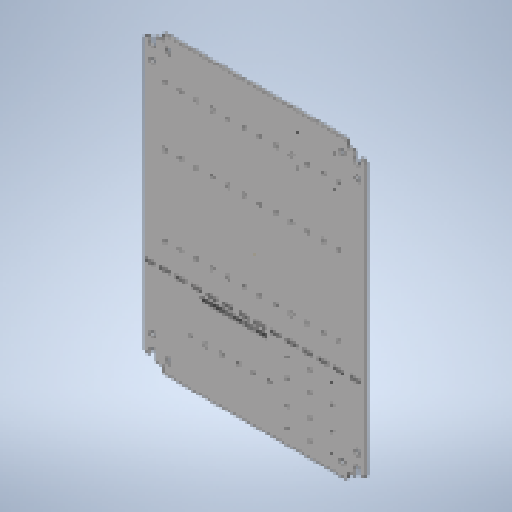
# Autodesk Inventor part: assembly-board
Saved by Autodesk Inventor 2023 (Build 270158030, 158C)
## iProperties
Created: 2024-03-20
Part Number: assembly-board
Material: Generic
Document SubType Name: Modeling
Designer: Imogen Heard
Density: 1 g/cm^3
Appearance: Default
Author: Imogen Heard
Autodesk Inventor part; units mm, degrees
(part 1 of 2)
ref_plane "YZ Plane" through (0, 0, 0) normal (1, 0, 0) x (0, 1, 0)
ref_plane "XZ Plane" through (0, 0, 0) normal (0, 1, 0) x (-1, 0, 0)
ref_plane "XY Plane" through (0, 0, 0) normal (0, 0, 1) x (1, 0, 0)
sketch "high voltage" plane through (0, 0, 0) normal (0, 0, 1) x (1, 0, 0)
  line L0 (-121.4929, -169.2156) -> (-167.7133, -169.2156)
  line L1 (-169.4454, -166.2156) -> (-146.3352, -126.1875)
  line L2 (-142.8711, -126.1875) -> (-119.7608, -166.2156)
  arc A0 (-142.8711, -126.1875) -> (-146.3352, -126.1875) centre (-144.6031, -127.1875) ccw
  arc A1 (-169.4454, -166.2156) -> (-167.7133, -169.2156) centre (-167.7133, -167.2156) ccw
  arc A2 (-121.4929, -169.2156) -> (-119.7608, -166.2156) centre (-121.4929, -167.2156) ccw
  line L3 (-145.4691, -126.6875) -> (-168.5793, -166.7156)
  arc A3 (-168.5793, -166.7156) -> (-167.7133, -168.2156) centre (-167.7133, -167.2156) ccw
  line L4 (-167.7133, -168.2156) -> (-121.4929, -168.2156)
  arc A4 (-121.4929, -168.2156) -> (-120.6269, -166.7156) centre (-121.4929, -167.2156) ccw
  line L5 (-120.6269, -166.7156) -> (-143.7371, -126.6875)
  arc A5 (-143.7371, -126.6875) -> (-145.4691, -126.6875) centre (-144.6031, -127.1875) ccw
  line L6 (-146.1782, -139.2847) -> (-142.8711, -139.2847)
  line L7 (-142.8711, -139.2847) -> (-147.4472, -150.1934)
  line L8 (-147.4472, -150.1934) -> (-140.7016, -147.4551)
  line L9 (-140.7016, -147.4551) -> (-144.0744, -160.167)
  line L10 (-144.0744, -160.167) -> (-142.8711, -160.167)
  line L11 (-142.8711, -160.167) -> (-145.822, -164.4859)
  line L12 (-145.822, -164.4859) -> (-147.4472, -160.0557)
  line L13 (-147.4472, -160.0557) -> (-146.1782, -160.0557)
  line L14 (-146.1782, -160.0557) -> (-143.8332, -151.8141)
  line L15 (-143.8332, -151.8141) -> (-150.3785, -154.471)
  line L16 (-150.3785, -154.471) -> (-146.1782, -139.2847)
  point P0 (-144.8622, -153.6861)
  point P1 (-144.6031, -153.8729)
  point P2 (-144.6031, -153.8729)
  point P3 (-118.0288, -169.2156)
  point P4 (-171.1774, -169.2156)
  point P5 (-144.6031, -123.1875)
  dimension "d142" = 2
  dimension "d146" = 1
  measures "d142" radius of A0
  measures "d146" distance between parallel lines of L3 L1
sketch "Sketch1" plane through (0, 0, 0) normal (0, 0, 1) x (1, 0, 0)
  line L0 (-175, 232.5) -> (175, 232.5)
  line L1 (175, 232.5) -> (175, -232.5)
  line L2 (175, -232.5) -> (-175, -232.5)
  line L3 (-175, -232.5) -> (-175, 232.5)
  point P0 (0, 0)
  dimension "d0" = 350
  dimension "d1" = 465
  dimension "d2" = 232.5
  dimension "d3" = 175
  constraints: 8 end point, 2 parallel, 1 horizontal, 1 perpendicular
  measures "d0" distance between parallel lines of L1 L3
  measures "d1" distance between parallel lines of L2 L0
  measures "d2" distance from line of point (0, 0) L0
  measures "d3" distance from line of point (0, 0) L1
extrude "Extrusion1" add sketch "Sketch1" along normal blind 3
sketch "Sketch3" plane through (0, 0, 3) normal (0, 0, 1) x (1, 0, 0)
  line L0 (-175, -232.5) -> (175, -232.5) projected
  line L1 (175, 232.5) -> (-175, 232.5) projected
  line L2 (175, -232.5) -> (175, 232.5) projected
  line L3 (-175, 232.5) -> (-175, -232.5) projected
  line L4 (-175, 232.5) -> (-146.5, 232.5)
  line L5 (-146.5, 232.5) -> (-146.5, 222.5)
  line L6 (-146.5, 222.5) -> (-175, 222.5)
  line L7 (-175, 222.5) -> (-175, 232.5)
  line L8 (-156, 216.5) -> (-175, 216.5)
  line L9 (-175, 216.5) -> (-175, 222.5)
  line L10 (-175, 222.5) -> (-156, 222.5)
  line L11 (-156, 222.5) -> (-156, 216.5)
  line L12 (-156, 216.5) -> (-167, 216.5)
  line L13 (-167, 216.5) -> (-167, 211.5)
  line L14 (-167, 211.5) -> (-156, 211.5)
  line L15 (-156, 211.5) -> (-156, 216.5)
  arc A0 (-167, 211.5) -> (-156, 211.5) centre (-161.5, 211.5) ccw
  line L16 (-146.5, 229.5) -> (-143.5, 232.5)
  line L17 (-175, 213.5) -> (-172, 216.5)
  circle A1 centre (-162, 187) radius 4.2
  circle A2 centre (-137.5, 211.5) radius 4.2
  point P0 (0, 0)
  dimension "d7" = 465
  dimension "d8" = 350
  dimension "d9" = 28.5
  dimension "d10" = 10
  dimension "d11" = 6
  dimension "d12" = 19
  dimension "d14" = 5
  dimension "d15" = 11
  dimension "d16" = 45
  dimension "d17" = 3
  dimension "d18" = 3
  dimension "d19" = 45
  dimension "d22" = 8.4
  dimension "d23" = 13
  dimension "d24" = 13.5
  dimension "d25" = 45.5
  dimension "d26" = 37.5
  dimension "d27" = 21
  constraints: 28 end point, 6 parallel, 3 centre point, 3 horizontal, 3 perpendicular, 3 point on line, 2 coincident, 2 point on circle, 1 equal radius, 1 horizontal alignment, 1 midpoint
  measures "d7" distance between parallel lines of L0 L1
  measures "d8" distance between parallel lines of L2 L3
  measures "d9" distance between parallel lines of L3 L5
  measures "d10" distance between parallel lines of L6 L1
  measures "d11" distance between parallel lines of L8 L6
  measures "d12" distance between parallel lines of L3 L11
  measures "d14" distance between parallel lines of L14 L12
  measures "d15" distance between parallel lines of L13 L15
  measures "d16" angle of L5 L16
  measures "d17" distance of L4.end L16.end
  measures "d18" distance from line of L3 L17.end
  measures "d19" angle of L8 L17
  measures "d22" diameter of A2
  measures "d23" distance from line of L3 A1.centre
  measures "d24" distance from line of L3 A0.centre
  measures "d25" distance from line of A1.centre L1
  measures "d26" distance from line of A2.centre L3
  measures "d27" distance from line of L1 A2.centre
extrude "Extrusion2" cut sketch "Sketch3" against normal through all contours L3 L8 L17 | L3 L6 L11 L8 | L16 L5 L1 | L3 L1 L5 L6 | L8 L15 L14 L13 | L14 A0 | A1 | A2
mirror "Mirror1" about plane through (0, 0, 0) normal (1, 0, 0) of "Extrusion2"
mirror "Mirror2" about plane through (0, 0, 0) normal (0, 1, 0) of "Extrusion2", "Mirror1"
sketch "Sketch4" plane through (0, 0, 3) normal (0, 0, 1) x (1, 0, 0)
  circle A0 centre (66.2112, 202.7338) radius 1.35 projected
  circle A1 centre (124.2112, 202.7338) radius 1.35 projected
  circle A2 centre (124.2112, 153.7338) radius 1.35 projected
  circle A3 centre (66.2112, 153.7338) radius 1.35 projected
  circle A4 centre (-142.425, 75.1905) radius 2.6
  arc A5 (113.375, 71.9905) -> (113.375, 78.3905) centre (113.375, 75.1905) ccw projected
  line L0 (113.375, 71.9905) -> (101.775, 71.9905) projected
  arc A6 (101.775, 78.3905) -> (101.775, 71.9905) centre (101.775, 75.1905) ccw projected
  line L1 (101.775, 78.3905) -> (113.375, 78.3905) projected
  arc A7 (-111.625, 71.9905) -> (-111.625, 78.3905) centre (-111.625, 75.1905) ccw projected
  line L2 (-111.625, 71.9905) -> (-123.225, 71.9905) projected
  arc A8 (-123.225, 78.3905) -> (-123.225, 71.9905) centre (-123.225, 75.1905) ccw projected
  line L3 (-123.225, 78.3905) -> (-111.625, 78.3905) projected
  arc A9 (13.375, 71.9905) -> (13.375, 78.3905) centre (13.375, 75.1905) ccw projected
  line L4 (13.375, 71.9905) -> (1.775, 71.9905) projected
  arc A10 (1.775, 78.3905) -> (1.775, 71.9905) centre (1.775, 75.1905) ccw projected
  line L5 (1.775, 78.3905) -> (13.375, 78.3905) projected
  arc A11 (-11.625, 71.9905) -> (-11.625, 78.3905) centre (-11.625, 75.1905) ccw projected
  line L6 (-11.625, 71.9905) -> (-23.225, 71.9905) projected
  arc A12 (-23.225, 78.3905) -> (-23.225, 71.9905) centre (-23.225, 75.1905) ccw projected
  line L7 (-23.225, 78.3905) -> (-11.625, 78.3905) projected
  arc A13 (-86.625, 71.9905) -> (-86.625, 78.3905) centre (-86.625, 75.1905) ccw projected
  line L8 (-86.625, 71.9905) -> (-98.225, 71.9905) projected
  arc A14 (-98.225, 78.3905) -> (-98.225, 71.9905) centre (-98.225, 75.1905) ccw projected
  line L9 (-98.225, 78.3905) -> (-86.625, 78.3905) projected
  arc A15 (88.375, 71.9905) -> (88.375, 78.3905) centre (88.375, 75.1905) ccw projected
  line L10 (88.375, 71.9905) -> (76.775, 71.9905) projected
  arc A16 (76.775, 78.3905) -> (76.775, 71.9905) centre (76.775, 75.1905) ccw projected
  line L11 (76.775, 78.3905) -> (88.375, 78.3905) projected
  arc A17 (138.375, 71.9905) -> (138.375, 78.3905) centre (138.375, 75.1905) ccw projected
  line L12 (138.375, 71.9905) -> (126.775, 71.9905) projected
  arc A18 (126.775, 78.3905) -> (126.775, 71.9905) centre (126.775, 75.1905) ccw projected
  line L13 (126.775, 78.3905) -> (138.375, 78.3905) projected
  arc A19 (-61.625, 71.9905) -> (-61.625, 78.3905) centre (-61.625, 75.1905) ccw projected
  line L14 (-61.625, 71.9905) -> (-73.225, 71.9905) projected
  arc A20 (-73.225, 78.3905) -> (-73.225, 71.9905) centre (-73.225, 75.1905) ccw projected
  line L15 (-73.225, 78.3905) -> (-61.625, 78.3905) projected
  arc A21 (38.375, 71.9905) -> (38.375, 78.3905) centre (38.375, 75.1905) ccw projected
  line L16 (38.375, 71.9905) -> (26.775, 71.9905) projected
  arc A22 (26.775, 78.3905) -> (26.775, 71.9905) centre (26.775, 75.1905) ccw projected
  line L17 (26.775, 78.3905) -> (38.375, 78.3905) projected
  arc A23 (-36.625, 71.9905) -> (-36.625, 78.3905) centre (-36.625, 75.1905) ccw projected
  line L18 (-36.625, 71.9905) -> (-48.225, 71.9905) projected
  arc A24 (-48.225, 78.3905) -> (-48.225, 71.9905) centre (-48.225, 75.1905) ccw projected
  line L19 (-48.225, 78.3905) -> (-36.625, 78.3905) projected
  line L20 (-148.225, 78.3905) -> (-136.625, 78.3905) projected
  arc A25 (-136.625, 71.9905) -> (-136.625, 78.3905) centre (-136.625, 75.1905) ccw projected
  line L21 (-136.625, 71.9905) -> (-148.225, 71.9905) projected
  arc A26 (-148.225, 78.3905) -> (-148.225, 71.9905) centre (-148.225, 75.1905) ccw projected
  arc A27 (63.375, 71.9905) -> (63.375, 78.3905) centre (63.375, 75.1905) ccw projected
  line L22 (63.375, 71.9905) -> (51.775, 71.9905) projected
  arc A28 (51.775, 78.3905) -> (51.775, 71.9905) centre (51.775, 75.1905) ccw projected
  line L23 (51.775, 78.3905) -> (63.375, 78.3905) projected
  line L24 (-155.025, 86.8905) -> (-155.025, 63.4905) projected
  line L25 (-155.025, 63.4905) -> (144.975, 63.4905) projected
  line L26 (144.975, 86.8905) -> (144.975, 63.4905) projected
  line L27 (-155.025, 86.8905) -> (144.975, 86.8905) projected
  circle A29 centre (-117.425, 75.1905) radius 2.6
  circle A30 centre (-92.425, 75.1905) radius 2.6
  circle A31 centre (-67.425, 75.1905) radius 2.6
  circle A32 centre (-42.425, 75.1905) radius 2.6
  circle A33 centre (-17.425, 75.1905) radius 2.6
  circle A34 centre (7.575, 75.1905) radius 2.6
  circle A35 centre (32.575, 75.1905) radius 2.6
  circle A36 centre (57.575, 75.1905) radius 2.6
  circle A37 centre (82.575, 75.1905) radius 2.6
  circle A38 centre (107.575, 75.1905) radius 2.6
  circle A39 centre (132.575, 75.1905) radius 2.6
  circle A40 centre (-142.425, -49.8095) radius 2.6
  circle A41 centre (-117.425, -49.8095) radius 2.6
  circle A42 centre (-92.425, -49.8095) radius 2.6
  circle A43 centre (-67.425, -49.8095) radius 2.6
  circle A44 centre (-42.425, -49.8095) radius 2.6
  circle A45 centre (-17.425, -49.8095) radius 2.6
  circle A46 centre (7.575, -49.8095) radius 2.6
  circle A47 centre (32.575, -49.8095) radius 2.6
  circle A48 centre (57.575, -49.8095) radius 2.6
  circle A49 centre (82.575, -49.8095) radius 2.6
  circle A50 centre (107.575, -49.8095) radius 2.6
  circle A51 centre (132.575, -49.8095) radius 2.6
  line L28 (24.975, -156.6095) -> (24.975, -148.1095) projected
  line L29 (-115.025, -148.1095) -> (24.975, -148.1095) projected
  line L30 (-115.025, -148.1095) -> (-115.025, -171.5095) projected
  line L31 (-115.025, -171.5095) -> (24.975, -171.5095) projected
  line L32 (24.975, -171.5095) -> (24.975, -163.0095) projected
  line L33 (24.975, -163.0095) -> (16.775, -163.0095) projected
  arc A52 (16.775, -156.6095) -> (16.775, -163.0095) centre (16.775, -159.8095) ccw projected
  line L34 (16.775, -156.6095) -> (24.975, -156.6095) projected
  arc A53 (-71.625, -163.0095) -> (-71.625, -156.6095) centre (-71.625, -159.8095) ccw projected
  line L35 (-71.625, -163.0095) -> (-83.225, -163.0095) projected
  arc A54 (-83.225, -156.6095) -> (-83.225, -163.0095) centre (-83.225, -159.8095) ccw projected
  line L36 (-83.225, -156.6095) -> (-71.625, -156.6095) projected
  arc A55 (-46.625, -163.0095) -> (-46.625, -156.6095) centre (-46.625, -159.8095) ccw projected
  line L37 (-46.625, -163.0095) -> (-58.225, -163.0095) projected
  arc A56 (-58.225, -156.6095) -> (-58.225, -163.0095) centre (-58.225, -159.8095) ccw projected
  line L38 (-58.225, -156.6095) -> (-46.625, -156.6095) projected
  arc A57 (-21.625, -163.0095) -> (-21.625, -156.6095) centre (-21.625, -159.8095) ccw projected
  line L39 (-21.625, -163.0095) -> (-33.225, -163.0095) projected
  arc A58 (-33.225, -156.6095) -> (-33.225, -163.0095) centre (-33.225, -159.8095) ccw projected
  line L40 (-33.225, -156.6095) -> (-21.625, -156.6095) projected
  arc A59 (3.375, -163.0095) -> (3.375, -156.6095) centre (3.375, -159.8095) ccw projected
  line L41 (3.375, -163.0095) -> (-8.225, -163.0095) projected
  arc A60 (-8.225, -156.6095) -> (-8.225, -163.0095) centre (-8.225, -159.8095) ccw projected
  line L42 (-8.225, -156.6095) -> (3.375, -156.6095) projected
  line L43 (-108.225, -156.6095) -> (-96.625, -156.6095) projected
  arc A61 (-96.625, -163.0095) -> (-96.625, -156.6095) centre (-96.625, -159.8095) ccw projected
  line L44 (-96.625, -163.0095) -> (-108.225, -163.0095) projected
  arc A62 (-108.225, -156.6095) -> (-108.225, -163.0095) centre (-108.225, -159.8095) ccw projected
  circle A63 centre (-102.425, -159.8095) radius 2.6
  circle A64 centre (-77.425, -159.8095) radius 2.6
  circle A65 centre (-52.425, -159.8095) radius 2.6
  circle A66 centre (-27.425, -159.8095) radius 2.6
  circle A67 centre (-2.425, -159.8095) radius 2.6
  circle A68 centre (22.575, -159.8095) radius 2.6
  arc A69 (49.282, -111.3926) -> (52.922, -111.3926) centre (51.102, -111.3926) ccw projected
  arc A70 (84.282, -111.3926) -> (87.922, -111.3926) centre (86.102, -111.3926) ccw projected
  arc A71 (119.282, -111.3926) -> (122.922, -111.3926) centre (121.102, -111.3926) ccw projected
  circle A72 centre (121.102, -142.2926) radius 1.82 projected
  circle A73 centre (86.102, -142.2926) radius 1.82 projected
  circle A74 centre (51.102, -142.2926) radius 1.82 projected
  circle A75 centre (51.102, -178.1926) radius 1.82 projected
  circle A76 centre (86.102, -178.1926) radius 1.82 projected
  circle A77 centre (121.102, -178.1926) radius 1.82 projected
  arc A78 (122.922, -209.0926) -> (119.282, -209.0926) centre (121.102, -209.0926) ccw projected
  arc A79 (87.922, -209.0926) -> (84.282, -209.0926) centre (86.102, -209.0926) ccw projected
  arc A80 (52.922, -209.0926) -> (49.282, -209.0926) centre (51.102, -209.0926) ccw projected
  circle A81 centre (51.102, -209.0926) radius 1.6
  circle A82 centre (86.102, -209.0926) radius 1.6
  circle A83 centre (121.102, -209.0926) radius 1.6
  circle A84 centre (51.102, -111.5926) radius 1.6
  circle A85 centre (86.102, -111.5926) radius 1.6
  circle A86 centre (121.102, -111.5926) radius 1.6
  circle A87 centre (-142.425, 167.1905) radius 2.6
  circle A88 centre (-117.425, 75.1905) radius 2.6
  circle A89 centre (-117.425, 167.1905) radius 2.6
  circle A90 centre (-92.425, 75.1905) radius 2.6
  circle A91 centre (-92.425, 167.1905) radius 2.6
  circle A92 centre (-67.425, 75.1905) radius 2.6
  circle A93 centre (-67.425, 167.1905) radius 2.6
  circle A94 centre (-42.425, 75.1905) radius 2.6
  circle A95 centre (-42.425, 167.1905) radius 2.6
  circle A96 centre (-17.425, 75.1905) radius 2.6
  circle A97 centre (-17.425, 167.1905) radius 2.6
  circle A98 centre (7.575, 75.1905) radius 2.6
  circle A99 centre (7.575, 167.1905) radius 2.6
  circle A100 centre (32.575, 75.1905) radius 2.6
  circle A101 centre (32.575, 167.1905) radius 2.6
  circle A102 centre (57.575, 75.1905) radius 2.6
  circle A103 centre (57.575, 167.1905) radius 2.6
  circle A104 centre (82.575, 75.1905) radius 2.6
  circle A105 centre (82.575, 167.1905) radius 2.6
  circle A106 centre (107.575, 75.1905) radius 2.6
  circle A107 centre (107.575, 167.1905) radius 2.6
  circle A108 centre (132.575, 75.1905) radius 2.6
  circle A109 centre (132.575, 167.1905) radius 2.6
  point P0 (0, 0)
  dimension "d28" = 5.2
  dimension "d29" = 5.8
  dimension "d30" = 5.8
  dimension "d31" = 25
  dimension "d34" = 25
  dimension "d37" = 125
  dimension "d40" = 5.2
  dimension "d41" = 5.8
  dimension "d44" = 25
  dimension "d49" = 3.2
  dimension "d52" = 35
  dimension "d55" = 97.5
  dimension "d60" = 92
  dimension "d63" = 25
  constraints: 59 centre point, 4 horizontal, 3 vertical, 2 horizontal alignment, 1 coincident, 112 other
  measures "d28" diameter of A4
  measures "d29" distance of A26.centre A4.centre
  measures "d30" distance of A25.centre A4.centre
  measures "d31" distance of A7.centre A25.centre
  measures "d34" distance of A4.centre A29.centre
  measures "d37" distance of A4.centre A40.centre
  measures "d40" diameter of A63
  measures "d41" distance of A62.centre A63.centre
  measures "d44" distance of A63.centre A64.centre
  measures "d49" diameter of A81
  measures "d52" distance of A81.centre A82.centre
  measures "d55" distance of A81.centre A84.centre
  measures "d60" distance of A4.centre A87.centre
  measures "d63" distance of A4.centre A88.centre
extrude "Extrusion3" cut sketch "Sketch4" against normal through all contours A0 | A1 | A2 | A3 | A4 | A29 | A30 | A31 | A32 | A33 | A34 | A35 | A36 | A37 | A38 | A39 | A40 | A41 | A42 | A43 | A44 | A45 | A46 | A47 | A48 | A49 | A50 | A51 | A63 | A64 | A65 | A66 | A67 | A68 | A72 | A73 | A74 | A75 | A76 | A77 | A81 | A82 | A83 | A84 | A85 | A86 | A87 | A89 | A91 | A93 | A95 | A97 | A99 | A101 | A103 | A105 | A107 | A109
sketch "Sketch5" plane through (0, 0, 3) normal (0, 0, 1) x (1, 0, 0)
  line L0 (-175, 213.5) -> (-175, -213.5) projected
  line L1 (-175, -87.5) -> (-160, -87.5)
  line L2 (-160, -87.5) -> (-160, -91.5)
  line L3 (-160, -91.5) -> (-175, -91.5)
  line L4 (-175, -91.5) -> (-175, -87.5)
  line L5 (-143.5, -232.5) -> (143.5, -232.5) projected
  line L6 (-150, -87.5) -> (-135, -87.5)
  line L7 (-135, -91.5) -> (-150, -91.5)
  line L8 (-135, -87.5) -> (-135, -91.5)
  line L9 (-150, -91.5) -> (-150, -87.5)
  line L10 (-125, -87.5) -> (-110, -87.5)
  line L11 (-110, -91.5) -> (-125, -91.5)
  line L12 (-110, -87.5) -> (-110, -91.5)
  line L13 (-125, -91.5) -> (-125, -87.5)
  line L14 (-100, -87.5) -> (-85, -87.5)
  line L15 (-85, -91.5) -> (-100, -91.5)
  line L16 (-85, -87.5) -> (-85, -91.5)
  line L17 (-100, -91.5) -> (-100, -87.5)
  line L18 (-75, -87.5) -> (-60, -87.5)
  line L19 (-60, -91.5) -> (-75, -91.5)
  line L20 (-60, -87.5) -> (-60, -91.5)
  line L21 (-75, -91.5) -> (-75, -87.5)
  line L22 (-50, -87.5) -> (-35, -87.5)
  line L23 (-35, -91.5) -> (-50, -91.5)
  line L24 (-35, -87.5) -> (-35, -91.5)
  line L25 (-50, -91.5) -> (-50, -87.5)
  line L26 (-25, -87.5) -> (-10, -87.5)
  line L27 (-10, -91.5) -> (-25, -91.5)
  line L28 (-10, -87.5) -> (-10, -91.5)
  line L29 (-25, -91.5) -> (-25, -87.5)
  line L30 (0, -87.5) -> (15, -87.5)
  line L31 (15, -91.5) -> (0, -91.5)
  line L32 (15, -87.5) -> (15, -91.5)
  line L33 (0, -91.5) -> (0, -87.5)
  line L34 (25, -87.5) -> (40, -87.5)
  line L35 (40, -91.5) -> (25, -91.5)
  line L36 (40, -87.5) -> (40, -91.5)
  line L37 (25, -91.5) -> (25, -87.5)
  line L38 (50, -87.5) -> (65, -87.5)
  line L39 (65, -91.5) -> (50, -91.5)
  line L40 (65, -87.5) -> (65, -91.5)
  line L41 (50, -91.5) -> (50, -87.5)
  line L42 (75, -91.5) -> (75, -87.5)
  line L43 (90, -91.5) -> (75, -91.5)
  line L44 (90, -87.5) -> (90, -91.5)
  line L45 (75, -87.5) -> (90, -87.5)
  line L46 (100, -91.5) -> (100, -87.5)
  line L47 (115, -91.5) -> (100, -91.5)
  line L48 (115, -87.5) -> (115, -91.5)
  line L49 (100, -87.5) -> (115, -87.5)
  line L50 (125, -91.5) -> (125, -87.5)
  line L51 (140, -91.5) -> (125, -91.5)
  line L52 (140, -87.5) -> (140, -91.5)
  line L53 (125, -87.5) -> (140, -87.5)
  line L54 (150, -91.5) -> (150, -87.5)
  line L55 (165, -91.5) -> (150, -91.5)
  line L56 (165, -87.5) -> (165, -91.5)
  line L57 (150, -87.5) -> (165, -87.5)
  line L58 (-84.5169, -96.4994) -> (24.8633, -96.4994) construction
  line L59 (24.8633, -96.4994) -> (24.8633, -107.8996) construction
  line L60 (24.8633, -107.8996) -> (-84.5169, -107.8996) construction
  line L61 (-84.5169, -107.8996) -> (-84.5169, -96.4994) construction
  line L62 (-67.4562, -118.0258) -> (-47.9562, -118.0258)
  line L63 (-47.9562, -118.0258) -> (-47.9562, -203.2928)
  line L64 (-47.9562, -203.2928) -> (-67.4562, -203.2928)
  line L65 (-67.4562, -203.2928) -> (-67.4562, -118.0258)
  line L66 (-48.9562, -202.2928) -> (-48.9562, -119.0258)
  line L67 (-48.9562, -119.0258) -> (-66.4562, -119.0258)
  line L68 (-66.4562, -119.0258) -> (-66.4562, -202.2928)
  line L69 (-66.4562, -202.2928) -> (-48.9562, -202.2928)
  line L70 (-29.4562, -119.0258) -> (-46.9562, -119.0258)
  line L71 (-47.9562, -118.0258) -> (-28.4562, -118.0258)
  line L72 (-29.4562, -202.2928) -> (-29.4562, -119.0258)
  line L73 (-46.9562, -119.0258) -> (-46.9562, -202.2928)
  line L74 (-28.4562, -118.0258) -> (-28.4562, -203.2928)
  line L75 (-46.9562, -202.2928) -> (-29.4562, -202.2928)
  line L76 (-28.4562, -203.2928) -> (-47.9562, -203.2928)
  line L77 (-47.9562, -203.2928) -> (-47.9562, -118.0258)
  line L78 (-9.9562, -119.0258) -> (-27.4562, -119.0258)
  line L79 (-28.4562, -118.0258) -> (-8.9562, -118.0258)
  line L80 (-9.9562, -202.2928) -> (-9.9562, -119.0258)
  line L81 (-27.4562, -119.0258) -> (-27.4562, -202.2928)
  line L82 (-8.9562, -118.0258) -> (-8.9562, -203.2928)
  line L83 (-27.4562, -202.2928) -> (-9.9562, -202.2928)
  line L84 (-8.9562, -203.2928) -> (-28.4562, -203.2928)
  line L85 (-28.4562, -203.2928) -> (-28.4562, -118.0258)
  line L86 (9.5438, -119.0258) -> (-7.9562, -119.0258)
  line L87 (-8.9562, -118.0258) -> (10.5438, -118.0258)
  line L88 (9.5438, -202.2928) -> (9.5438, -119.0258)
  line L89 (-7.9562, -119.0258) -> (-7.9562, -202.2928)
  line L90 (10.5438, -118.0258) -> (10.5438, -203.2928)
  line L91 (-7.9562, -202.2928) -> (9.5438, -202.2928)
  line L92 (10.5438, -203.2928) -> (-8.9562, -203.2928)
  line L93 (-8.9562, -203.2928) -> (-8.9562, -118.0258)
  line L94 (29.0438, -119.0258) -> (11.5438, -119.0258)
  line L95 (10.5438, -118.0258) -> (30.0438, -118.0258)
  line L96 (29.0438, -202.2928) -> (29.0438, -119.0258)
  line L97 (11.5438, -119.0258) -> (11.5438, -202.2928)
  line L98 (30.0438, -118.0258) -> (30.0438, -203.2928)
  line L99 (11.5438, -202.2928) -> (29.0438, -202.2928)
  line L100 (30.0438, -203.2928) -> (10.5438, -203.2928)
  line L101 (10.5438, -203.2928) -> (10.5438, -118.0258)
  line L102 (-59.7232, -120.1793) -> (-51.7369, -120.1793) construction
  line L103 (-51.7369, -120.1793) -> (-51.7369, -126.2793) construction
  line L104 (-51.7369, -126.2793) -> (-59.7232, -126.2793) construction
  line L105 (-59.7232, -126.2793) -> (-59.7232, -120.1793) construction
  line L106 (-42.5354, -120.1793) -> (-31.6524, -120.1793) construction
  line L107 (-31.6524, -120.1793) -> (-31.6524, -126.2793) construction
  line L108 (-31.6524, -126.2793) -> (-42.5354, -126.2793) construction
  line L109 (-42.5354, -126.2793) -> (-42.5354, -120.1793) construction
  line L110 (-3.0255, -126.2793) -> (-3.0255, -120.1793) construction
  line L111 (-3.0255, -120.1793) -> (5.8128, -120.1793) construction
  line L112 (5.8128, -120.1793) -> (5.8128, -126.2793) construction
  line L113 (5.8128, -126.2793) -> (-3.0255, -126.2793) construction
  line L114 (-22.6436, -126.2793) -> (-22.6436, -120.1793) construction
  line L115 (-22.6436, -120.1793) -> (-13.8054, -120.1793) construction
  line L116 (-13.8054, -120.1793) -> (-13.8054, -126.2793) construction
  line L117 (-13.8054, -126.2793) -> (-22.6436, -126.2793) construction
  line L118 (16.0367, -126.2793) -> (16.0367, -120.1793) construction
  line L119 (16.0367, -120.1793) -> (24.8749, -120.1793) construction
  line L120 (24.8749, -120.1793) -> (24.8749, -126.2793) construction
  line L121 (24.8749, -126.2793) -> (16.0367, -126.2793) construction
  line L122 (-110, 10.5365) -> (-60, 10.5365)
  line L123 (-60, 10.5365) -> (-60, -84.0099)
  line L124 (-60, -84.0099) -> (-110, -84.0099)
  line L125 (-110, -84.0099) -> (-110, 10.5365)
  line L126 (-60, 10.5365) -> (2, 10.5365)
  line L127 (2, 10.5365) -> (2, -84.0099)
  line L128 (2, -84.0099) -> (-60, -84.0099)
  line L129 (-60, -84.0099) -> (-60, 10.5365)
  line L130 (2, 10.5365) -> (22, 10.5365)
  line L131 (22, 10.5365) -> (22, -84.0099)
  line L132 (22, -84.0099) -> (2, -84.0099)
  line L133 (2, -84.0099) -> (2, 10.5365)
  line L134 (-61, 9.5365) -> (-109, 9.5365)
  line L135 (-109, 9.5365) -> (-109, -83.0099)
  line L136 (-109, -83.0099) -> (-61, -83.0099)
  line L137 (-61, -83.0099) -> (-61, 9.5365)
  line L138 (3, 9.5365) -> (21, 9.5365)
  line L139 (21, 9.5365) -> (21, -83.0099)
  line L140 (21, -83.0099) -> (3, -83.0099)
  line L141 (3, -83.0099) -> (3, 9.5365)
  line L142 (-59, 9.5365) -> (1, 9.5365)
  line L143 (1, 9.5365) -> (1, -83.0099)
  line L144 (1, -83.0099) -> (-59, -83.0099)
  line L145 (-59, -83.0099) -> (-59, 9.5365)
  line L146 (-91.3061, 0.557) -> (-91.3061, 6.657) construction
  line L147 (-91.3061, 6.657) -> (-75.4153, 6.657) construction
  line L148 (-75.4153, 6.657) -> (-75.4153, 0.557) construction
  line L149 (-75.4153, 0.557) -> (-91.3061, 0.557) construction
  line L150 (-37.021, 0.7734) -> (-37.021, 6.8734) construction
  line L151 (-37.021, 6.8734) -> (-21.1303, 6.8734) construction
  line L152 (-21.1303, 6.8734) -> (-21.1303, 0.7734) construction
  line L153 (-21.1303, 0.7734) -> (-37.021, 0.7734) construction
  line L154 (3.7464, 2.4981) -> (3.7464, 8.5981) construction
  line L155 (3.7464, 8.5981) -> (19.6371, 8.5981) construction
  line L156 (19.6371, 8.5981) -> (19.6371, 2.4981) construction
  line L157 (19.6371, 2.4981) -> (3.7464, 2.4981) construction
  line L158 (-124.5738, -162.6593) -> (-170.7943, -162.6593)
  line L159 (-172.5263, -159.6593) -> (-149.4161, -119.6312)
  line L160 (-145.952, -119.6312) -> (-122.8418, -159.6593)
  arc A0 (-145.952, -119.6312) -> (-149.4161, -119.6312) centre (-147.6841, -120.6312) ccw
  arc A1 (-172.5263, -159.6593) -> (-170.7943, -162.6593) centre (-170.7943, -160.6593) ccw
  arc A2 (-124.5738, -162.6593) -> (-122.8418, -159.6593) centre (-124.5738, -160.6593) ccw
  line L161 (-148.5501, -120.1312) -> (-171.6603, -160.1593)
  arc A3 (-171.6603, -160.1593) -> (-170.7943, -161.6593) centre (-170.7943, -160.6593) ccw
  line L162 (-170.7943, -161.6593) -> (-124.5738, -161.6593)
  arc A4 (-124.5738, -161.6593) -> (-123.7078, -160.1593) centre (-124.5738, -160.6593) ccw
  line L163 (-123.7078, -160.1593) -> (-146.818, -120.1312)
  arc A5 (-146.818, -120.1312) -> (-148.5501, -120.1312) centre (-147.6841, -120.6312) ccw
  line L164 (-149.2591, -132.7285) -> (-145.952, -132.7285)
  line L165 (-145.952, -132.7285) -> (-150.5281, -143.6371)
  line L166 (-150.5281, -143.6371) -> (-143.7825, -140.8988)
  line L167 (-143.7825, -140.8988) -> (-147.1553, -153.6108)
  line L168 (-147.1553, -153.6108) -> (-145.952, -153.6108)
  line L169 (-145.952, -153.6108) -> (-148.9029, -157.9297)
  line L170 (-148.9029, -157.9297) -> (-150.5281, -153.4994)
  line L171 (-150.5281, -153.4994) -> (-149.2591, -153.4994)
  line L172 (-149.2591, -153.4994) -> (-146.9142, -145.2578)
  line L173 (-146.9142, -145.2578) -> (-153.4594, -147.9148)
  line L174 (-153.4594, -147.9148) -> (-149.2591, -132.7285)
  line L175 (-77.0625, -96.6279) -> (-78.5949, -102.7279)
  line L176 (-78.5949, -102.7279) -> (-79.5044, -102.7279)
  line L177 (-79.5044, -102.7279) -> (-80.7452, -97.666)
  line L178 (-80.7452, -97.666) -> (-81.9514, -102.7279)
  line L179 (-81.9514, -102.7279) -> (-82.851, -102.7279)
  line L180 (-82.851, -102.7279) -> (-84.4082, -96.6279)
  line L181 (-84.4082, -96.6279) -> (-83.5727, -96.6279)
  line L182 (-83.5727, -96.6279) -> (-82.3468, -101.6849)
  line L183 (-82.3468, -101.6849) -> (-81.1308, -96.6279)
  line L184 (-81.1308, -96.6279) -> (-80.3052, -96.6279)
  line L185 (-80.3052, -96.6279) -> (-79.0793, -101.7442)
  line L186 (-79.0793, -101.7442) -> (-77.8583, -96.6279)
  line L187 (-77.8583, -96.6279) -> (-77.0625, -96.6279)
  line L188 (-76.9933, -102.7279) -> (-74.9368, -96.6279)
  line L189 (-74.9368, -96.6279) -> (-73.9383, -96.6279)
  line L190 (-73.9383, -96.6279) -> (-71.8819, -102.7279)
  line L191 (-71.8819, -102.7279) -> (-72.7371, -102.7279)
  line L192 (-72.7371, -102.7279) -> (-73.2907, -101.0225)
  line L193 (-73.2907, -101.0225) -> (-75.619, -101.0225)
  line L194 (-75.619, -101.0225) -> (-76.1727, -102.7279)
  line L195 (-76.1727, -102.7279) -> (-76.9933, -102.7279)
  line L196 (-73.5132, -100.3304) -> (-74.4574, -97.4584)
  line L197 (-74.4574, -97.4584) -> (-75.3966, -100.3304)
  line L198 (-75.3966, -100.3304) -> (-73.5132, -100.3304)
  line L199 (-66.5827, -102.7279) -> (-67.6356, -102.7279)
  line L200 (-67.6356, -102.7279) -> (-69.5635, -100.3007)
  line L201 (-69.5635, -100.3007) -> (-70.4928, -100.3007)
  line L202 (-70.4928, -100.3007) -> (-70.4928, -102.7279)
  line L203 (-70.4928, -102.7279) -> (-71.3035, -102.7279)
  line L204 (-71.3035, -102.7279) -> (-71.3035, -96.6279)
  line L205 (-71.3035, -96.6279) -> (-69.7316, -96.6279)
  spline S0 degree 2 poles (-69.7316, -96.6279) (-69.2076, -96.6279) (-68.5007, -96.7416) (-68.1794, -96.9492) knots 0 0 0 1 2 2 2
  spline S1 degree 2 poles (-68.1794, -96.9492) (-67.8581, -97.1568) (-67.4873, -97.8044) (-67.4873, -98.2839) knots 0 0 0 1 2 2 2
  spline S2 degree 2 poles (-67.4873, -98.2839) (-67.4873, -98.9512) (-68.1695, -99.8559) (-68.7528, -100.0734) knots 0 0 0 1 2 2 2
  line L206 (-68.7528, -100.0734) -> (-66.5827, -102.7279)
  spline S3 degree 2 poles (-68.3326, -98.3482) (-68.3326, -98.0812) (-68.5205, -97.6709) (-68.7182, -97.5375) knots 0 0 0 1 2 2 2
  spline S4 degree 2 poles (-68.7182, -97.5375) (-68.8912, -97.4238) (-69.3509, -97.3298) (-69.6871, -97.3298) knots 0 0 0 1 2 2 2
  line L207 (-69.6871, -97.3298) -> (-70.4928, -97.3298)
  line L208 (-70.4928, -97.3298) -> (-70.4928, -99.6235)
  line L209 (-70.4928, -99.6235) -> (-69.781, -99.6235)
  spline S5 degree 2 poles (-69.781, -99.6235) (-69.43, -99.6235) (-68.8715, -99.4999) (-68.6787, -99.3071) knots 0 0 0 1 2 2 2
  spline S6 degree 2 poles (-68.6787, -99.3071) (-68.5007, -99.1391) (-68.3326, -98.6645) (-68.3326, -98.3482) knots 0 0 0 1 2 2 2
  line L210 (-61.7334, -102.7279) -> (-62.6429, -102.7279)
  line L211 (-62.6429, -102.7279) -> (-65.342, -97.4682)
  line L212 (-65.342, -97.4682) -> (-65.342, -102.7279)
  line L213 (-65.342, -102.7279) -> (-66.0983, -102.7279)
  line L214 (-66.0983, -102.7279) -> (-66.0983, -96.6279)
  line L215 (-66.0983, -96.6279) -> (-64.9465, -96.6279)
  line L216 (-64.9465, -96.6279) -> (-62.4897, -101.4575)
  line L217 (-62.4897, -101.4575) -> (-62.4897, -96.6279)
  line L218 (-62.4897, -96.6279) -> (-61.7334, -96.6279)
  line L219 (-61.7334, -96.6279) -> (-61.7334, -102.7279)
  line L220 (-58.3719, -102.7279) -> (-60.7348, -102.7279)
  line L221 (-60.7348, -102.7279) -> (-60.7348, -102.105)
  line L222 (-60.7348, -102.105) -> (-59.9587, -102.105)
  line L223 (-59.9587, -102.105) -> (-59.9587, -97.2507)
  line L224 (-59.9587, -97.2507) -> (-60.7348, -97.2507)
  line L225 (-60.7348, -97.2507) -> (-60.7348, -96.6279)
  line L226 (-60.7348, -96.6279) -> (-58.3719, -96.6279)
  line L227 (-58.3719, -96.6279) -> (-58.3719, -97.2507)
  line L228 (-58.3719, -97.2507) -> (-59.148, -97.2507)
  line L229 (-59.148, -97.2507) -> (-59.148, -102.105)
  line L230 (-59.148, -102.105) -> (-58.3719, -102.105)
  line L231 (-58.3719, -102.105) -> (-58.3719, -102.7279)
  line L232 (-53.0035, -102.7279) -> (-53.9131, -102.7279)
  line L233 (-53.9131, -102.7279) -> (-56.6121, -97.4682)
  line L234 (-56.6121, -97.4682) -> (-56.6121, -102.7279)
  line L235 (-56.6121, -102.7279) -> (-57.3685, -102.7279)
  line L236 (-57.3685, -102.7279) -> (-57.3685, -96.6279)
  line L237 (-57.3685, -96.6279) -> (-56.2167, -96.6279)
  line L238 (-56.2167, -96.6279) -> (-53.7599, -101.4575)
  line L239 (-53.7599, -101.4575) -> (-53.7599, -96.6279)
  line L240 (-53.7599, -96.6279) -> (-53.0035, -96.6279)
  line L241 (-53.0035, -96.6279) -> (-53.0035, -102.7279)
  spline S7 degree 2 poles (-49.2121, -102.8465) (-49.8596, -102.8465) (-50.9323, -102.4511) (-51.3179, -102.0507) knots 0 0 0 1 2 2 2
  spline S8 degree 2 poles (-51.3179, -102.0507) (-51.7035, -101.6453) (-52.1138, -100.449) (-52.1138, -99.6729) knots 0 0 0 1 2 2 2
  spline S9 degree 2 poles (-52.1138, -99.6729) (-52.1138, -98.9364) (-51.6985, -97.7698) (-51.3129, -97.3546) knots 0 0 0 1 2 2 2
  spline S10 degree 2 poles (-51.3129, -97.3546) (-50.9422, -96.9541) (-49.8547, -96.5191) (-49.2071, -96.5191) knots 0 0 0 1 2 2 2
  spline S11 degree 2 poles (-49.2071, -96.5191) (-48.8957, -96.5191) (-48.3321, -96.6081) (-48.0751, -96.6872) knots 0 0 0 1 2 2 2
  spline S12 degree 2 poles (-48.0751, -96.6872) (-47.8675, -96.7465) (-47.3633, -96.964) (-47.21, -97.0431) knots 0 0 0 1 2 2 2
  line L242 (-47.21, -97.0431) -> (-47.21, -98.0219)
  line L243 (-47.21, -98.0219) -> (-47.2792, -98.0219)
  spline S13 degree 2 poles (-47.2792, -98.0219) (-47.4325, -97.8884) (-47.7538, -97.6462) (-48.0504, -97.5078) knots 0 0 0 1 2 2 2
  spline S14 degree 2 poles (-48.0504, -97.5078) (-48.2975, -97.3842) (-48.9352, -97.2211) (-49.301, -97.2211) knots 0 0 0 1 2 2 2
  spline S15 degree 2 poles (-49.301, -97.2211) (-50.1809, -97.2211) (-51.2685, -98.5459) (-51.2685, -99.6482) knots 0 0 0 1 2 2 2
  spline S16 degree 2 poles (-51.2685, -99.6482) (-51.2685, -100.2612) (-50.9817, -101.1806) (-50.7099, -101.497) knots 0 0 0 1 2 2 2
  spline S17 degree 2 poles (-50.7099, -101.497) (-50.4479, -101.8134) (-49.7064, -102.1446) (-49.2417, -102.1446) knots 0 0 0 1 2 2 2
  spline S18 degree 2 poles (-49.2417, -102.1446) (-48.9006, -102.1446) (-48.2185, -102.0457) (-47.9861, -101.9469) knots 0 0 0 1 2 2 2
  line L244 (-47.9861, -101.9469) -> (-47.9861, -100.37)
  line L245 (-47.9861, -100.37) -> (-49.3999, -100.37)
  line L246 (-49.3999, -100.37) -> (-49.3999, -99.6581)
  line L247 (-49.3999, -99.6581) -> (-47.1853, -99.6581)
  line L248 (-47.1853, -99.6581) -> (-47.1853, -102.3225)
  spline S19 degree 2 poles (-47.1853, -102.3225) (-47.3386, -102.3917) (-47.8625, -102.6043) (-48.085, -102.6686) knots 0 0 0 1 2 2 2
  spline S20 degree 2 poles (-48.085, -102.6686) (-48.3865, -102.7576) (-48.871, -102.8465) (-49.2121, -102.8465) knots 0 0 0 1 2 2 2
  line L249 (-44.8125, -102.7279) -> (-45.7913, -102.7279)
  line L250 (-45.7913, -102.7279) -> (-45.7913, -101.5613)
  line L251 (-45.7913, -101.5613) -> (-44.8125, -101.5613)
  line L252 (-44.8125, -101.5613) -> (-44.8125, -102.7279)
  line L253 (-44.8125, -99.317) -> (-45.7913, -99.317)
  line L254 (-45.7913, -99.317) -> (-45.7913, -98.1504)
  line L255 (-45.7913, -98.1504) -> (-44.8125, -98.1504)
  line L256 (-44.8125, -98.1504) -> (-44.8125, -99.317)
  line L257 (-36.1519, -102.7279) -> (-36.9626, -102.7279)
  line L258 (-36.9626, -102.7279) -> (-36.9626, -99.7422)
  line L259 (-36.9626, -99.7422) -> (-39.7704, -99.7422)
  line L260 (-39.7704, -99.7422) -> (-39.7704, -102.7279)
  line L261 (-39.7704, -102.7279) -> (-40.5811, -102.7279)
  line L262 (-40.5811, -102.7279) -> (-40.5811, -96.6279)
  line L263 (-40.5811, -96.6279) -> (-39.7704, -96.6279)
  line L264 (-39.7704, -96.6279) -> (-39.7704, -99.0204)
  line L265 (-39.7704, -99.0204) -> (-36.9626, -99.0204)
  line L266 (-36.9626, -99.0204) -> (-36.9626, -96.6279)
  line L267 (-36.9626, -96.6279) -> (-36.1519, -96.6279)
  line L268 (-36.1519, -96.6279) -> (-36.1519, -102.7279)
  line L269 (-32.7905, -102.7279) -> (-35.1534, -102.7279)
  line L270 (-35.1534, -102.7279) -> (-35.1534, -102.105)
  line L271 (-35.1534, -102.105) -> (-34.3773, -102.105)
  line L272 (-34.3773, -102.105) -> (-34.3773, -97.2507)
  line L273 (-34.3773, -97.2507) -> (-35.1534, -97.2507)
  line L274 (-35.1534, -97.2507) -> (-35.1534, -96.6279)
  line L275 (-35.1534, -96.6279) -> (-32.7905, -96.6279)
  line L276 (-32.7905, -96.6279) -> (-32.7905, -97.2507)
  line L277 (-32.7905, -97.2507) -> (-33.5666, -97.2507)
  line L278 (-33.5666, -97.2507) -> (-33.5666, -102.105)
  line L279 (-33.5666, -102.105) -> (-32.7905, -102.105)
  line L280 (-32.7905, -102.105) -> (-32.7905, -102.7279)
  spline S21 degree 2 poles (-29.2313, -102.8465) (-29.8789, -102.8465) (-30.9516, -102.4511) (-31.3372, -102.0507) knots 0 0 0 1 2 2 2
  spline S22 degree 2 poles (-31.3372, -102.0507) (-31.7227, -101.6453) (-32.133, -100.449) (-32.133, -99.6729) knots 0 0 0 1 2 2 2
  spline S23 degree 2 poles (-32.133, -99.6729) (-32.133, -98.9364) (-31.7178, -97.7698) (-31.3322, -97.3546) knots 0 0 0 1 2 2 2
  spline S24 degree 2 poles (-31.3322, -97.3546) (-30.9615, -96.9541) (-29.874, -96.5191) (-29.2264, -96.5191) knots 0 0 0 1 2 2 2
  spline S25 degree 2 poles (-29.2264, -96.5191) (-28.915, -96.5191) (-28.3514, -96.6081) (-28.0944, -96.6872) knots 0 0 0 1 2 2 2
  spline S26 degree 2 poles (-28.0944, -96.6872) (-27.8868, -96.7465) (-27.3826, -96.964) (-27.2293, -97.0431) knots 0 0 0 1 2 2 2
  line L281 (-27.2293, -97.0431) -> (-27.2293, -98.0219)
  line L282 (-27.2293, -98.0219) -> (-27.2985, -98.0219)
  spline S27 degree 2 poles (-27.2985, -98.0219) (-27.4518, -97.8884) (-27.7731, -97.6462) (-28.0697, -97.5078) knots 0 0 0 1 2 2 2
  spline S28 degree 2 poles (-28.0697, -97.5078) (-28.3168, -97.3842) (-28.9545, -97.2211) (-29.3203, -97.2211) knots 0 0 0 1 2 2 2
  spline S29 degree 2 poles (-29.3203, -97.2211) (-30.2002, -97.2211) (-31.2877, -98.5459) (-31.2877, -99.6482) knots 0 0 0 1 2 2 2
  spline S30 degree 2 poles (-31.2877, -99.6482) (-31.2877, -100.2612) (-31.001, -101.1806) (-30.7291, -101.497) knots 0 0 0 1 2 2 2
  spline S31 degree 2 poles (-30.7291, -101.497) (-30.4672, -101.8134) (-29.7257, -102.1446) (-29.261, -102.1446) knots 0 0 0 1 2 2 2
  spline S32 degree 2 poles (-29.261, -102.1446) (-28.9199, -102.1446) (-28.2377, -102.0457) (-28.0054, -101.9469) knots 0 0 0 1 2 2 2
  line L283 (-28.0054, -101.9469) -> (-28.0054, -100.37)
  line L284 (-28.0054, -100.37) -> (-29.4192, -100.37)
  line L285 (-29.4192, -100.37) -> (-29.4192, -99.6581)
  line L286 (-29.4192, -99.6581) -> (-27.2046, -99.6581)
  line L287 (-27.2046, -99.6581) -> (-27.2046, -102.3225)
  spline S33 degree 2 poles (-27.2046, -102.3225) (-27.3578, -102.3917) (-27.8818, -102.6043) (-28.1043, -102.6686) knots 0 0 0 1 2 2 2
  spline S34 degree 2 poles (-28.1043, -102.6686) (-28.4058, -102.7576) (-28.8903, -102.8465) (-29.2313, -102.8465) knots 0 0 0 1 2 2 2
  line L288 (-21.7571, -102.7279) -> (-22.5678, -102.7279)
  line L289 (-22.5678, -102.7279) -> (-22.5678, -99.7422)
  line L290 (-22.5678, -99.7422) -> (-25.3756, -99.7422)
  line L291 (-25.3756, -99.7422) -> (-25.3756, -102.7279)
  line L292 (-25.3756, -102.7279) -> (-26.1863, -102.7279)
  line L293 (-26.1863, -102.7279) -> (-26.1863, -96.6279)
  line L294 (-26.1863, -96.6279) -> (-25.3756, -96.6279)
  line L295 (-25.3756, -96.6279) -> (-25.3756, -99.0204)
  line L296 (-25.3756, -99.0204) -> (-22.5678, -99.0204)
  line L297 (-22.5678, -99.0204) -> (-22.5678, -96.6279)
  line L298 (-22.5678, -96.6279) -> (-21.7571, -96.6279)
  line L299 (-21.7571, -96.6279) -> (-21.7571, -102.7279)
  line L300 (-13.4771, -96.6279) -> (-15.578, -102.7279)
  line L301 (-15.578, -102.7279) -> (-16.453, -102.7279)
  line L302 (-16.453, -102.7279) -> (-18.5539, -96.6279)
  line L303 (-18.5539, -96.6279) -> (-17.6838, -96.6279)
  line L304 (-17.6838, -96.6279) -> (-15.9932, -101.6947)
  line L305 (-15.9932, -101.6947) -> (-14.3026, -96.6279)
  line L306 (-14.3026, -96.6279) -> (-13.4771, -96.6279)
  spline S35 degree 2 poles (-8.5783, -97.3249) (-8.2323, -97.7302) (-7.8467, -98.9166) (-7.8467, -99.6779) knots 0 0 0 1 2 2 2
  spline S36 degree 2 poles (-7.8467, -99.6779) (-7.8467, -100.4194) (-8.2224, -101.6206) (-8.5783, -102.0259) knots 0 0 0 1 2 2 2
  spline S37 degree 2 poles (-8.5783, -102.0259) (-8.954, -102.4511) (-9.9476, -102.8564) (-10.5458, -102.8564) knots 0 0 0 1 2 2 2
  spline S38 degree 2 poles (-10.5458, -102.8564) (-11.1637, -102.8564) (-12.1523, -102.4362) (-12.5132, -102.0259) knots 0 0 0 1 2 2 2
  spline S39 degree 2 poles (-12.5132, -102.0259) (-12.8642, -101.6206) (-13.2398, -100.4293) (-13.2398, -99.6779) knots 0 0 0 1 2 2 2
  spline S40 degree 2 poles (-13.2398, -99.6779) (-13.2398, -98.9117) (-12.8592, -97.7451) (-12.5082, -97.3249) knots 0 0 0 1 2 2 2
  spline S41 degree 2 poles (-12.5082, -97.3249) (-12.1523, -96.9195) (-11.1587, -96.4994) (-10.5458, -96.4994) knots 0 0 0 1 2 2 2
  spline S42 degree 2 poles (-10.5458, -96.4994) (-9.9229, -96.4994) (-8.9244, -96.9344) (-8.5783, -97.3249) knots 0 0 0 1 2 2 2
  spline S43 degree 2 poles (-8.692, -99.6779) (-8.692, -99.0748) (-8.954, -98.1405) (-9.1913, -97.8341) knots 0 0 0 1 2 2 2
  spline S44 degree 2 poles (-9.1913, -97.8341) (-9.4335, -97.5177) (-10.1157, -97.2013) (-10.5408, -97.2013) knots 0 0 0 1 2 2 2
  spline S45 degree 2 poles (-10.5408, -97.2013) (-10.9808, -97.2013) (-11.6432, -97.5078) (-11.8953, -97.8341) knots 0 0 0 1 2 2 2
  spline S46 degree 2 poles (-11.8953, -97.8341) (-12.1375, -98.1455) (-12.3945, -99.0847) (-12.3945, -99.6779) knots 0 0 0 1 2 2 2
  spline S47 degree 2 poles (-12.3945, -99.6779) (-12.3945, -100.8791) (-11.3861, -102.1545) (-10.5408, -102.1545) knots 0 0 0 1 2 2 2
  spline S48 degree 2 poles (-10.5408, -102.1545) (-9.6955, -102.1545) (-8.692, -100.8791) (-8.692, -99.6779) knots 0 0 0 1 2 2 2
  line L307 (-3.4225, -102.7279) -> (-6.9569, -102.7279)
  line L308 (-6.9569, -102.7279) -> (-6.9569, -96.6279)
  line L309 (-6.9569, -96.6279) -> (-6.1462, -96.6279)
  line L310 (-6.1462, -96.6279) -> (-6.1462, -102.0062)
  line L311 (-6.1462, -102.0062) -> (-3.4225, -102.0062)
  line L312 (-3.4225, -102.0062) -> (-3.4225, -102.7279)
  line L313 (-1.3612, -102.7279) -> (-1.3612, -97.3496)
  line L314 (-1.3612, -97.3496) -> (-3.4077, -97.3496)
  line L315 (-3.4077, -97.3496) -> (-3.4077, -96.6279)
  line L316 (-3.4077, -96.6279) -> (1.4961, -96.6279)
  line L317 (1.4961, -96.6279) -> (1.4961, -97.3496)
  line L318 (1.4961, -97.3496) -> (-0.5505, -97.3496)
  line L319 (-0.5505, -97.3496) -> (-0.5505, -102.7279)
  line L320 (-0.5505, -102.7279) -> (-1.3612, -102.7279)
  line L321 (1.4565, -102.7279) -> (3.5129, -96.6279)
  line L322 (3.5129, -96.6279) -> (4.5115, -96.6279)
  line L323 (4.5115, -96.6279) -> (6.5679, -102.7279)
  line L324 (6.5679, -102.7279) -> (5.7127, -102.7279)
  line L325 (5.7127, -102.7279) -> (5.159, -101.0225)
  line L326 (5.159, -101.0225) -> (2.8307, -101.0225)
  line L327 (2.8307, -101.0225) -> (2.2771, -102.7279)
  line L328 (2.2771, -102.7279) -> (1.4565, -102.7279)
  line L329 (4.9366, -100.3304) -> (3.9924, -97.4584)
  line L330 (3.9924, -97.4584) -> (3.0532, -100.3304)
  line L331 (3.0532, -100.3304) -> (4.9366, -100.3304)
  spline S49 degree 2 poles (9.7019, -102.8465) (9.0543, -102.8465) (7.9816, -102.4511) (7.5961, -102.0507) knots 0 0 0 1 2 2 2
  spline S50 degree 2 poles (7.5961, -102.0507) (7.2105, -101.6453) (6.8002, -100.449) (6.8002, -99.6729) knots 0 0 0 1 2 2 2
  spline S51 degree 2 poles (6.8002, -99.6729) (6.8002, -98.9364) (7.2154, -97.7698) (7.601, -97.3546) knots 0 0 0 1 2 2 2
  spline S52 degree 2 poles (7.601, -97.3546) (7.9717, -96.9541) (9.0593, -96.5191) (9.7068, -96.5191) knots 0 0 0 1 2 2 2
  spline S53 degree 2 poles (9.7068, -96.5191) (10.0183, -96.5191) (10.5818, -96.6081) (10.8388, -96.6872) knots 0 0 0 1 2 2 2
  spline S54 degree 2 poles (10.8388, -96.6872) (11.0465, -96.7465) (11.5507, -96.964) (11.7039, -97.0431) knots 0 0 0 1 2 2 2
  line L332 (11.7039, -97.0431) -> (11.7039, -98.0219)
  line L333 (11.7039, -98.0219) -> (11.6347, -98.0219)
  spline S55 degree 2 poles (11.6347, -98.0219) (11.4815, -97.8884) (11.1602, -97.6462) (10.8636, -97.5078) knots 0 0 0 1 2 2 2
  spline S56 degree 2 poles (10.8636, -97.5078) (10.6164, -97.3842) (9.9787, -97.2211) (9.6129, -97.2211) knots 0 0 0 1 2 2 2
  spline S57 degree 2 poles (9.6129, -97.2211) (8.733, -97.2211) (7.6455, -98.5459) (7.6455, -99.6482) knots 0 0 0 1 2 2 2
  spline S58 degree 2 poles (7.6455, -99.6482) (7.6455, -100.2612) (7.9322, -101.1806) (8.2041, -101.497) knots 0 0 0 1 2 2 2
  spline S59 degree 2 poles (8.2041, -101.497) (8.4661, -101.8134) (9.2076, -102.1446) (9.6722, -102.1446) knots 0 0 0 1 2 2 2
  spline S60 degree 2 poles (9.6722, -102.1446) (10.0133, -102.1446) (10.6955, -102.0457) (10.9278, -101.9469) knots 0 0 0 1 2 2 2
  line L334 (10.9278, -101.9469) -> (10.9278, -100.37)
  line L335 (10.9278, -100.37) -> (9.514, -100.37)
  line L336 (9.514, -100.37) -> (9.514, -99.6581)
  line L337 (9.514, -99.6581) -> (11.7286, -99.6581)
  line L338 (11.7286, -99.6581) -> (11.7286, -102.3225)
  spline S61 degree 2 poles (11.7286, -102.3225) (11.5754, -102.3917) (11.0514, -102.6043) (10.829, -102.6686) knots 0 0 0 1 2 2 2
  spline S62 degree 2 poles (10.829, -102.6686) (10.5274, -102.7576) (10.043, -102.8465) (9.7019, -102.8465) knots 0 0 0 1 2 2 2
  line L339 (12.7469, -102.7279) -> (12.7469, -96.6279)
  line L340 (12.7469, -96.6279) -> (16.5632, -96.6279)
  line L341 (16.5632, -96.6279) -> (16.5632, -97.3496)
  line L342 (16.5632, -97.3496) -> (13.5576, -97.3496)
  line L343 (13.5576, -97.3496) -> (13.5576, -99.0204)
  line L344 (13.5576, -99.0204) -> (16.3605, -99.0204)
  line L345 (16.3605, -99.0204) -> (16.3605, -99.7422)
  line L346 (16.3605, -99.7422) -> (13.5576, -99.7422)
  line L347 (13.5576, -99.7422) -> (13.5576, -102.0062)
  line L348 (13.5576, -102.0062) -> (16.5632, -102.0062)
  line L349 (16.5632, -102.0062) -> (16.5632, -102.7279)
  line L350 (16.5632, -102.7279) -> (12.7469, -102.7279)
  line L351 (18.6838, -96.6279) -> (18.5701, -101.0472)
  line L352 (18.5701, -101.0472) -> (17.8929, -101.0472)
  line L353 (17.8929, -101.0472) -> (17.7693, -96.6279)
  line L354 (17.7693, -96.6279) -> (18.6838, -96.6279)
  line L355 (18.6443, -102.7279) -> (17.8089, -102.7279)
  line L356 (17.8089, -102.7279) -> (17.8089, -101.8628)
  line L357 (17.8089, -101.8628) -> (18.6443, -101.8628)
  line L358 (18.6443, -101.8628) -> (18.6443, -102.7279)
  spline S63 degree 2 poles (-38.0617, -122.0182) (-38.0617, -122.4137) (-38.3435, -123.1255) (-38.5956, -123.3727) knots 0 0 0 1 2 2 2
  spline S64 degree 2 poles (-38.5956, -123.3727) (-38.912, -123.6841) (-39.7672, -124.0054) (-40.4197, -124.0054) knots 0 0 0 1 2 2 2
  line L359 (-40.4197, -124.0054) -> (-41.1068, -124.0054)
  line L360 (-41.1068, -124.0054) -> (-41.1068, -126.2793)
  line L361 (-41.1068, -126.2793) -> (-41.9175, -126.2793)
  line L362 (-41.9175, -126.2793) -> (-41.9175, -120.1793)
  line L363 (-41.9175, -120.1793) -> (-40.3851, -120.1793)
  spline S65 degree 2 poles (-40.3851, -120.1793) (-39.8413, -120.1793) (-39.0801, -120.3573) (-38.7884, -120.5599) knots 0 0 0 1 2 2 2
  spline S66 degree 2 poles (-38.7884, -120.5599) (-38.4473, -120.7923) (-38.0617, -121.509) (-38.0617, -122.0182) knots 0 0 0 1 2 2 2
  spline S67 degree 2 poles (-38.907, -122.0429) (-38.907, -121.7265) (-39.1246, -121.2619) (-39.347, -121.1136) knots 0 0 0 1 2 2 2
  spline S68 degree 2 poles (-39.347, -121.1136) (-39.5398, -120.9851) (-40.0539, -120.8812) (-40.4345, -120.8812) knots 0 0 0 1 2 2 2
  line L364 (-40.4345, -120.8812) -> (-41.1068, -120.8812)
  line L365 (-41.1068, -120.8812) -> (-41.1068, -123.3133)
  line L366 (-41.1068, -123.3133) -> (-40.5532, -123.3133)
  spline S69 degree 2 poles (-40.5532, -123.3133) (-40.0588, -123.3133) (-39.4508, -123.1552) (-39.2531, -122.9475) knots 0 0 0 1 2 2 2
  spline S70 degree 2 poles (-39.2531, -122.9475) (-39.0702, -122.7646) (-38.907, -122.3346) (-38.907, -122.0429) knots 0 0 0 1 2 2 2
  line L367 (-37.2906, -126.2793) -> (-37.2906, -120.1793)
  line L368 (-37.2906, -120.1793) -> (-33.4744, -120.1793)
  line L369 (-33.4744, -120.1793) -> (-33.4744, -120.901)
  line L370 (-33.4744, -120.901) -> (-36.4799, -120.901)
  line L371 (-36.4799, -120.901) -> (-36.4799, -122.5718)
  line L372 (-36.4799, -122.5718) -> (-33.6771, -122.5718)
  line L373 (-33.6771, -122.5718) -> (-33.6771, -123.2936)
  line L374 (-33.6771, -123.2936) -> (-36.4799, -123.2936)
  line L375 (-36.4799, -123.2936) -> (-36.4799, -125.5576)
  line L376 (-36.4799, -125.5576) -> (-33.4744, -125.5576)
  line L377 (-33.4744, -125.5576) -> (-33.4744, -126.2793)
  line L378 (-33.4744, -126.2793) -> (-37.2906, -126.2793)
  line L379 (-54.7404, -126.2793) -> (-55.6499, -126.2793)
  line L380 (-55.6499, -126.2793) -> (-58.349, -121.0197)
  line L381 (-58.349, -121.0197) -> (-58.349, -126.2793)
  line L382 (-58.349, -126.2793) -> (-59.1053, -126.2793)
  line L383 (-59.1053, -126.2793) -> (-59.1053, -120.1793)
  line L384 (-59.1053, -120.1793) -> (-57.9535, -120.1793)
  line L385 (-57.9535, -120.1793) -> (-55.4967, -125.0089)
  line L386 (-55.4967, -125.0089) -> (-55.4967, -120.1793)
  line L387 (-55.4967, -120.1793) -> (-54.7404, -120.1793)
  line L388 (-54.7404, -120.1793) -> (-54.7404, -126.2793)
  line L389 (-18.4913, -126.2991) -> (-22.0257, -126.2991)
  line L390 (-22.0257, -126.2991) -> (-22.0257, -120.1991)
  line L391 (-22.0257, -120.1991) -> (-21.215, -120.1991)
  line L392 (-21.215, -120.1991) -> (-21.215, -125.5774)
  line L393 (-21.215, -125.5774) -> (-18.4913, -125.5774)
  line L394 (-18.4913, -125.5774) -> (-18.4913, -126.2991)
  line L395 (-14.5713, -126.2991) -> (-17.5471, -126.2991)
  line L396 (-17.5471, -126.2991) -> (-17.5471, -125.6762)
  line L397 (-17.5471, -125.6762) -> (-16.4398, -125.6762)
  line L398 (-16.4398, -125.6762) -> (-16.4398, -121.5881)
  line L399 (-16.4398, -121.5881) -> (-17.5471, -121.5881)
  line L400 (-17.5471, -121.5881) -> (-17.5471, -121.0295)
  spline S71 degree 2 poles (-17.5471, -121.0295) (-16.9193, -121.0295) (-16.3261, -120.6736) (-16.2866, -120.1793) knots 0 0 0 1 2 2 2
  line L401 (-16.2866, -120.1793) -> (-15.6539, -120.1793)
  line L402 (-15.6539, -120.1793) -> (-15.6539, -125.6762)
  line L403 (-15.6539, -125.6762) -> (-14.5713, -125.6762)
  line L404 (-14.5713, -125.6762) -> (-14.5713, -126.2991)
  line L405 (1.1268, -126.4078) -> (-2.4076, -126.4078)
  line L406 (-2.4076, -126.4078) -> (-2.4076, -120.3078)
  line L407 (-2.4076, -120.3078) -> (-1.5969, -120.3078)
  line L408 (-1.5969, -120.3078) -> (-1.5969, -125.6861)
  line L409 (-1.5969, -125.6861) -> (1.1268, -125.6861)
  line L410 (1.1268, -125.6861) -> (1.1268, -126.4078)
  line L411 (5.3533, -126.4078) -> (1.5915, -126.4078)
  line L412 (1.5915, -126.4078) -> (1.5915, -125.5428)
  spline S72 degree 2 poles (1.5915, -125.5428) (1.9969, -125.1621) (2.7186, -124.4552) (3.0646, -124.0746) knots 0 0 0 1 2 2 2